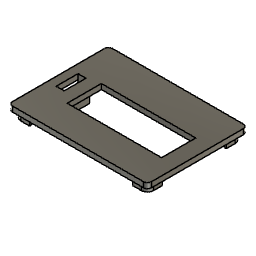
couvercle (Autodesk Fusion 360 design; units mm, degrees)
Autodesk Fusion 360 part; units mm, degrees
sketch "Esquisse1" plane through (0, 0, 0) normal (0, 0, 1) x (1, 0, 0)
  line L0 (102.7, 76) -> (3, 76)
  line L1 (0, 73) -> (0, 3)
  arc A0 (3, 76) -> (0, 73) centre (3, 73) ccw
  arc A1 (0, 3) -> (3, 0) centre (3, 3) ccw
  arc A2 (105.7, 73) -> (102.7, 76) centre (102.7, 73) ccw
  line L2 (6.5, 46.3) -> (12.55, 46.3)
  line L3 (12.55, 46.3) -> (12.55, 29.7)
  line L4 (12.55, 29.7) -> (6.5, 29.7)
  line L5 (6.5, 29.7) -> (6.5, 46.3)
  line L6 (21.9, 22.7) -> (93.7, 22.7)
  line L7 (93.7, 22.7) -> (93.7, 48.7)
  line L8 (93.7, 48.7) -> (21.9, 48.7)
  line L9 (21.9, 48.7) -> (21.9, 22.7)
  line L10 (12.55, 46.3) -> (6.5, 46.3)
  line L11 (6.5, 46.3) -> (6.5, 48.1)
  line L12 (6.5, 48.1) -> (12.55, 48.1)
  line L13 (12.55, 48.1) -> (12.55, 46.3)
  line L14 (12.55, 29.7) -> (6.5, 29.7)
  line L15 (6.5, 29.7) -> (6.5, 27.9)
  line L16 (6.5, 27.9) -> (12.55, 27.9)
  line L17 (12.55, 27.9) -> (12.55, 29.7)
  line L18 (2, 62) -> (1.9999, 62)
  line L19 (105.7, 73) -> (105.7, 3)
  arc A3 (102.7, 0) -> (105.7, 3) centre (102.7, 3) ccw
  line L20 (12.55, 27.9) -> (13.55, 27.9)
  line L21 (13.55, 27.9) -> (13.55, 48.1)
  line L22 (13.55, 48.1) -> (12.55, 48.1)
  line L23 (12.55, 48.1) -> (12.55, 27.9)
  line L24 (2, 14) -> (2, 7)
  line L25 (7, 2) -> (14, 2)
  arc A4 (2, 7) -> (7, 2) centre (7, 7) ccw
  line L26 (2, 14) -> (4, 14)
  line L27 (4, 14) -> (4, 7)
  line L28 (7, 4) -> (14, 4)
  line L29 (14, 2) -> (14, 4)
  arc A5 (4, 7) -> (7, 4) centre (7, 7) ccw
  line L30 (13.67, 2.33) -> (13.67, 3.67)
  line L31 (7, 3.67) -> (13.67, 3.67)
  arc A6 (3.67, 7) -> (7, 3.67) centre (7, 7) ccw
  line L32 (3.67, 13.67) -> (3.67, 7)
  line L33 (2.33, 13.67) -> (3.67, 13.67)
  line L34 (2.33, 13.67) -> (2.33, 7)
  arc A7 (2.33, 7) -> (7, 2.33) centre (7, 7) ccw
  line L35 (7, 2.33) -> (13.67, 2.33)
  line L36 (91.7, 2) -> (98.7, 2)
  line L37 (103.7, 7) -> (103.7, 14)
  line L38 (103.7, 14) -> (101.7, 14)
  line L39 (101.7, 14) -> (101.7, 7)
  line L40 (98.7, 4) -> (91.7, 4)
  line L41 (91.7, 4) -> (91.7, 2)
  arc A8 (98.7, 2) -> (103.7, 7) centre (98.7, 7) ccw
  arc A9 (98.7, 4) -> (101.7, 7) centre (98.7, 7) ccw
  line L42 (92.03, 2.33) -> (98.7, 2.33)
  arc A10 (98.7, 2.33) -> (103.37, 7) centre (98.7, 7) ccw
  line L43 (103.37, 7) -> (103.37, 13.67)
  line L44 (103.37, 13.67) -> (102.03, 13.67)
  line L45 (102.03, 13.67) -> (102.03, 7)
  arc A11 (98.7, 3.67) -> (102.03, 7) centre (98.7, 7) ccw
  line L46 (98.7, 3.67) -> (92.03, 3.67)
  line L47 (92.03, 3.67) -> (92.03, 2.33)
  line L48 (3, 0) -> (102.7, 0)
  line L49 (103.7, 62) -> (103.7, 69)
  line L50 (98.7, 74) -> (91.7, 74)
  line L51 (91.7, 74) -> (91.7, 72)
  line L52 (91.7, 72) -> (98.7, 72)
  line L53 (101.7, 69) -> (101.7, 62)
  line L54 (101.7, 62) -> (103.7, 62)
  arc A12 (101.7, 69) -> (98.7, 72) centre (98.7, 69) ccw
  arc A13 (103.7, 69) -> (98.7, 74) centre (98.7, 69) ccw
  line L55 (92.03, 72.33) -> (98.7, 72.33)
  arc A14 (102.03, 69) -> (98.7, 72.33) centre (98.7, 69) ccw
  line L56 (102.03, 69) -> (102.03, 62.33)
  line L57 (102.03, 62.33) -> (103.37, 62.33)
  line L58 (103.37, 62.33) -> (103.37, 69)
  arc A15 (103.37, 69) -> (98.7, 73.67) centre (98.7, 69) ccw
  line L59 (98.7, 73.67) -> (92.03, 73.67)
  line L60 (92.03, 73.67) -> (92.03, 72.33)
  line L61 (2, 62) -> (2, 69)
  line L62 (7, 74) -> (14, 74)
  line L63 (14, 74) -> (14, 72)
  line L64 (14, 72) -> (7, 72)
  line L65 (4, 69) -> (4, 62)
  line L66 (4, 62) -> (2, 62)
  arc A16 (7, 74) -> (2, 69) centre (7, 69) ccw
  arc A17 (7, 72) -> (4, 69) centre (7, 69) ccw
  line L67 (2.33, 62.33) -> (2.33, 69)
  arc A18 (7, 73.67) -> (2.33, 69) centre (7, 69) ccw
  line L68 (7, 73.67) -> (13.67, 73.67)
  line L69 (13.67, 73.67) -> (13.67, 72.33)
  line L70 (13.67, 72.33) -> (7, 72.33)
  arc A19 (7, 72.33) -> (3.67, 69) centre (7, 69) ccw
  line L71 (3.67, 69) -> (3.67, 62.33)
  line L72 (3.67, 62.33) -> (2.33, 62.33)
  point P0 (0, 76)
  point P1 (103.7, 2)
  point P2 (103.7, 74)
  point P3 (2, 74)
  dimension "d2" = 76
  dimension "d3" = 3
  dimension "d4" = 3
  dimension "d5" = 3
  dimension "d31" = 6.05
  dimension "d32" = 16.6
  dimension "d49" = 26
  dimension "d50" = 71.8
  dimension "d51" = 27.3
  dimension "d53" = 29.7
  dimension "d55" = 1.8
  dimension "d56" = 1.8
  dimension "d72" = 21.9
  dimension "d92" = 6.5
  dimension "d107" = 3
  dimension "d108" = 105.7
  dimension "d109" = 12
  dimension "d137" = 1
  dimension "d147" = 2
  dimension "d148" = 5
  dimension "d149" = 2
  dimension "d150" = 3
  dimension "d151" = 12
  dimension "d152" = 12
  dimension "d153" = -0.33
  dimension "d154" = 12
  dimension "d155" = 12
  dimension "d160" = 2
  dimension "d162" = 2
  dimension "d164" = 5
  dimension "d165" = 3
  dimension "d166" = -0.33
  dimension "d167" = 12
  dimension "d168" = 12
  dimension "d169" = 2
  dimension "d171" = 2
  dimension "d172" = 2
  dimension "d173" = 2
  dimension "d174" = 2
  dimension "d175" = 3
  dimension "d176" = 5
  dimension "d177" = -0.33
  dimension "d178" = 12
  dimension "d179" = 12
  dimension "d180" = 2
  dimension "d183" = 2
  dimension "d184" = 2
  dimension "d185" = 2
  dimension "d186" = 5
  dimension "d187" = 3
  dimension "d188" = -0.33
  constraint vertical L1
  constraint coincident P0 L0
  constraint coincident P0 L1
  constraint tangent L0 A0
  constraint tangent L1 A0
  constraint horizontal L2
  constraint vertical L3
  constraint horizontal L4
  constraint vertical L5
  constraint horizontal L6
  constraint vertical L7
  constraint horizontal L8
  constraint vertical L9
  constraint horizontal L10
  constraint vertical L11
  constraint horizontal L12
  constraint vertical L13
  constraint horizontal L14
  constraint vertical L15
  constraint horizontal L16
  constraint vertical L17
  constraint horizontal L20
  constraint vertical L21
  constraint horizontal L22
  constraint vertical L23
  constraint vertical L24
  constraint perpendicular L24 L25
  constraint tangent L24 A4
  constraint tangent L25 A4
  constraint perpendicular L24 L26
  constraint perpendicular L26 L27
  constraint perpendicular L24 L28
  constraint perpendicular L28 L29
  constraint tangent L27 A5
  constraint tangent L28 A5
  constraint horizontal L36
  constraint perpendicular L36 L37
  constraint perpendicular L37 L38
  constraint perpendicular L36 L39
  constraint perpendicular L39 L40
  constraint perpendicular L36 L41
  constraint coincident P1 L36
  constraint coincident P1 L37
  constraint tangent L36 A8
  constraint tangent L37 A8
  constraint tangent L39 A9
  constraint tangent L40 A9
  constraint tangent A3 L48
  constraint parallel L19 L49
  constraint perpendicular L19 L50
  constraint perpendicular L50 L51
  constraint perpendicular L19 L52
  constraint perpendicular L52 L53
  constraint perpendicular L49 L54
  constraint tangent L52 A12
  constraint tangent L53 A12
  constraint coincident P2 L49
  constraint coincident P2 L50
  constraint tangent L49 A13
  constraint tangent L50 A13
  constraint vertical L61
  constraint perpendicular L61 L62
  constraint perpendicular L62 L63
  constraint perpendicular L63 L64
  constraint perpendicular L62 L65
  constraint perpendicular L61 L66
  constraint coincident P3 L61
  constraint coincident P3 L62
  constraint tangent L61 A16
  constraint tangent L62 A16
  constraint tangent L64 A17
  constraint tangent L65 A17
  measures "d2" distance of origin P0
  measures "d3" radius of A0
  measures "d4" radius of A1
  measures "d5" radius of A2
  measures "d31" distance of L2.start L2.end
  measures "d32" distance of L2.start L4.end
  measures "d49" distance of L6.end L7.end
  measures "d50" distance of L7 L9
  measures "d51" distance of L0 L8
  measures "d53" distance of L0 L2
  measures "d55" distance of L10 L12
  measures "d56" distance of L14 L16
  measures "d72" distance of L1 L9
  measures "d92" distance of L1 L5
  measures "d107" radius of A3
  measures "d108" distance of L1 L19
  measures "d109" distance of L7 L19
  measures "d137" distance of L16.end L20.end
  measures "d147" distance of L1 L24
  measures "d148" radius of A4
  measures "d149" distance of L24.start L26.end
  measures "d150" radius of A5
  measures "d151" distance of L25 L26
  measures "d152" distance of L24 L29
  measures "d154" distance of L36.start P1
  measures "d155" distance of P1 L37.end
  measures "d160" distance of L37.end L38.end
  measures "d162" distance of L19 L37
  measures "d164" radius of A8
  measures "d165" radius of A9
  measures "d167" distance of L49.start P2
  measures "d168" distance of P2 L50.end
  measures "d169" distance of L50.end L51.end
  measures "d171" distance of L0 L50
  measures "d172" distance of L19 L49
  measures "d173" distance of L49.start L53.end
  measures "d174" distance of L36.start L40.end
  measures "d175" radius of A12
  measures "d176" radius of A13
  measures "d178" distance of L18.start P3
  measures "d179" distance of P3 L62.end
  measures "d180" distance of L62.end L63.end
  measures "d183" distance of L18.start L65.end
  measures "d184" distance of L0 L62
  measures "d185" distance of L1 L61
  measures "d186" radius of A16
  measures "d187" radius of A17
extrude "Extrusion1" add sketch "Esquisse1" against normal blind 4 contours L0 L1 A0 A1 A2 L19 A3 L48 | L24 L25 A4 L26 L27 L28 L29 A5 | L36 L37 L38 L39 L40 L41 A8 A9 | L49 L50 L51 L52 L53 L54 A12 A13 | L61 L62 L63 L64 L65 L66 A16 A17
extrude "Extrusion5" add sketch "Esquisse1" against normal blind 17 contours L2 L10 L11 L12 L13 L23 | L3 L13 L17 L20 L21 L22 L23 | L4 L14 L15 L16 L17 L23
extrude "Extrusion17" add sketch "Esquisse1" against normal blind 9 contours L30 L31 A6 L32 L33 L34 A7 L35 | L42 A10 L43 L44 L45 A11 L46 L47 | L55 A14 L56 L57 L58 A15 L59 L60 | L67 A18 L68 L69 L70 A19 L71 L72
equation "d36 = 17.55 mm - 3 mm"
equation "d41 = d32 - 0 mm"
equation "d53 = ( d2 - d32 ) / 2"
equation "d56 = d55"
equation "d158 = 12 mm"
equation "d159 = d158"
equation "d78 = 4.197624 mm"
equation "d79 = 8.198 mm"
equation "d80 = 8.208 mm"
equation "d81 = 6.207952 mm"
equation "d85 = 12 mm"
equation "d87 = -0.4 mm"
equation "d97 = d78"
equation "d98 = d79"
equation "d100 = d81"
equation "d103 = d87"
equation "d104 = d85"
equation "d112 = d80"
equation "d146 = 2 mm"
equation "d147 = d146"
equation "d152 = d151"
equation "d166 = d153"
equation "d177 = d166"
equation "d188 = d153"
equation "d189 = -4 mm - 5 mm"
